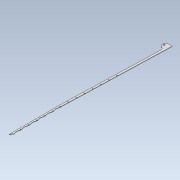
# Autodesk Inventor part: traverse_cote
Saved by Autodesk Inventor 2020 (Build 240168000, 168)
## iProperties
Created: 2020-09-10
Part Number: traverse_cote
Material: Generic
Document SubType Name: Modeling
Designer: Admin
Density: 1 g/cm^3
Appearance: Default
Author: Admin
Autodesk Inventor part; units mm, degrees
ref_plane "YZ Plane" through (0, 0, 0) normal (1, 0, 0) x (0, 1, 0)
ref_plane "XZ Plane" through (0, 0, 0) normal (0, 1, 0) x (-1, 0, 0)
ref_plane "XY Plane" through (0, 0, 0) normal (0, 0, 1) x (1, 0, 0)
sketch "Sketch1" plane through (0, 0, 0) normal (0, 1, 0) x (-1, 0, 0)
  line L0 (0, 0) -> (26.5, 0)
  line L1 (26.5, 0) -> (26.5, -260)
  line L2 (26.5, -260) -> (10, -800)
  line L3 (10, -800) -> (0, -800)
  line L4 (0, 0) -> (0, -10)
  line L5 (0, -10) -> (16.5, -10)
  line L6 (16.5, -10) -> (16.5, -260)
  line L7 (16.5, -260) -> (0, -800)
  dimension "d1" = 26.5
  dimension "d2" = 10
  dimension "d3" = 260
  dimension "d4" = 10
  dimension "d6" = 10
  dimension "d7" = 250
  dimension "d8" = 0
  dimension "d9" = 800
  constraints: 16 end point, 3 perpendicular, 1 coincident, 1 horizontal, 1 parallel, 1 vertical
  measures "d1" distance of L0.start L0.end
  measures "d2" distance of L2.end L3.end
  measures "d3" distance of L0.end L1.end
  measures "d4" distance of L0.start L4.end
  measures "d6" distance between parallel lines of L1 L6
  measures "d7" distance of L5.end L6.end
  measures "d8" horizontal distance of point (0, 0) L3.end
  measures "d9" distance between parallel lines of L0 L3
extrude "Extrusion1" add sketch "Sketch1" along normal mid plane 2
sketch "Sketch2" plane through (0, 1, 0) normal (0, 1, 0) x (1, 0, 0)
  line L0 (-21.5, 50) -> (0, 50)
  line L1 (0, 50) -> (0, 52)
  line L2 (0, 52) -> (-21.5, 52)
  line L3 (-21.5, 52) -> (-21.5, 50)
  line L4 (0, 0) -> (0, 10) projected
  line L5 (0, 10) -> (-16.5, 10) projected
  dimension "d12" = 2
  dimension "d13" = 21.5
  dimension "d14" = 0
  dimension "d16" = 40
  constraints: 8 end point, 2 parallel, 1 horizontal, 1 perpendicular
  measures "d12" distance of L2.end L0.start
  measures "d13" distance of L0.start L0.end
  measures "d14" distance between parallel lines of L4 L1
  measures "d16" distance between parallel lines of L0 L5
extrude "Extrusion2" cut sketch "Sketch2" against normal through all
pattern_linear "Rectangular Pattern1" count 6 spacing 40 along (0, 0, -1) of "Extrusion2"
sketch "Sketch3" plane through (0, 1, 0) normal (0, 1, 0) x (1, 0, 0)
  line L0 (-21.6, 290) -> (0, 290)
  line L1 (0, 290) -> (0, 292)
  line L2 (0, 292) -> (-21.6, 292)
  line L3 (-21.6, 292) -> (-21.6, 290)
  line L4 (0, 0) -> (0, 10) projected
  line L5 (-16.5, 250) -> (-21.5, 250) projected
  line L6 (-19.4, 330) -> (0, 330)
  line L7 (0, 330) -> (0, 332)
  line L8 (0, 332) -> (-19.4, 332)
  line L9 (-19.4, 332) -> (-19.4, 330)
  line L10 (-18.2, 370) -> (0, 370)
  line L11 (0, 370) -> (0, 372)
  line L12 (0, 372) -> (-18.2, 372)
  line L13 (-18.2, 372) -> (-18.2, 370)
  line L14 (-17, 410) -> (0, 410)
  line L15 (0, 410) -> (0, 412)
  line L16 (0, 412) -> (-17, 412)
  line L17 (-17, 412) -> (-17, 410)
  line L18 (-15.8, 450) -> (0, 450)
  line L19 (0, 450) -> (0, 452)
  line L20 (0, 452) -> (-15.8, 452)
  line L21 (-15.8, 452) -> (-15.8, 450)
  line L22 (-14.6, 490) -> (0, 490)
  line L23 (0, 490) -> (0, 492)
  line L24 (0, 492) -> (-14.6, 492)
  line L25 (-14.6, 492) -> (-14.6, 490)
  line L26 (-13.4, 530) -> (0, 530)
  line L27 (0, 530) -> (0, 532)
  line L28 (0, 532) -> (-13.4, 532)
  line L29 (-13.4, 532) -> (-13.4, 530)
  point P0 (-26.5, 250)
  dimension "d22" = 2
  dimension "d23" = 0
  dimension "d24" = 40
  dimension "d25" = 21.6
  dimension "d84" = 40
  dimension "d85" = 2
  dimension "d86" = 0
  dimension "d87" = 19.4
  dimension "d88" = 40
  dimension "d89" = 2
  dimension "d90" = 0
  dimension "d91" = 18.2
  dimension "d92" = 40
  dimension "d93" = 2
  dimension "d94" = 0
  dimension "d95" = 17
  dimension "d96" = 40
  dimension "d97" = 2
  dimension "d98" = 0
  dimension "d99" = 15.8
  dimension "d100" = 40
  dimension "d101" = 2
  dimension "d102" = 0
  dimension "d103" = 14.6
  dimension "d104" = 40
  dimension "d105" = 2
  dimension "d106" = 13.4
  dimension "d107" = 0
  constraints: 56 end point, 14 parallel, 7 horizontal, 7 perpendicular
  measures "d22" distance of L2.end L0.start
  measures "d23" distance from line of L4 L1.end
  measures "d24" distance between parallel lines of L5 L0
  measures "d25" distance of L1.end L2.end
  measures "d84" distance between parallel lines of L6 L0
  measures "d85" distance of L6.end L7.end
  measures "d86" distance between parallel lines of L1 L7
  measures "d87" distance of L6.start L6.end
  measures "d88" distance between parallel lines of L10 L6
  measures "d89" distance of L12.end L10.start
  measures "d90" distance between parallel lines of L7 L11
  measures "d91" distance of L10.start L10.end
  measures "d92" distance between parallel lines of L14 L10
  measures "d93" distance of L16.end L14.start
  measures "d94" distance from line of L10.end L15
  measures "d95" distance of L14.start L14.end
  measures "d96" distance between parallel lines of L18 L14
  measures "d97" distance of L20.end L18.start
  measures "d98" distance between parallel lines of L15 L19
  measures "d99" distance of L18.start L18.end
  measures "d100" distance between parallel lines of L22 L18
  measures "d101" distance of L24.end L22.start
  measures "d102" distance between parallel lines of L23 L19
  measures "d103" distance of L22.start L22.end
  measures "d104" distance between parallel lines of L22 L26
  measures "d105" distance of L28.end L26.start
  measures "d106" distance of L26.start L26.end
  measures "d107" distance from line of L27.end L23
extrude "Extrusion3" cut sketch "Sketch3" against normal through all
sketch "Sketch11" plane through (0, 1, 0) normal (0, 1, 0) x (1, 0, 0)
  line L0 (-22.25, 0) -> (0, 0)
  line L1 (0, 0) -> (0, 10)
  line L2 (0, 10) -> (-22.25, 10)
  line L3 (-22.25, 0) -> (-22.25, 7.5)
  line L4 (-22.25, 7.5) -> (-24.75, 7.5)
  line L5 (-24.75, 7.5) -> (-24.75, 10)
  line L6 (-24.75, 10) -> (-22.25, 10)
  dimension "d108" = 2.5
  dimension "d110" = 2.5
  dimension "d111" = 10
  dimension "d112" = 24.75
  constraints: 14 end point, 4 perpendicular, 1 coincident, 1 horizontal, 1 parallel, 1 point on line, 1 vertical
  measures "d108" distance of L4.end L5.end
  measures "d110" distance of L3.end L4.end
  measures "d111" distance of L0.end L1.end
  measures "d112" distance between parallel lines of L1 L5
extrude "Extrusion11" cut sketch "Sketch11" against normal blind 10
sketch "Sketch12" plane through (0, 1, 0) normal (0, 1, 0) x (1, 0, 0)
  line L0 (-24.75, 7.5) -> (-24.75, 10) projected
  line L1 (-24.75, 7.5) -> (-22.25, 7.5)
  line L2 (-22.25, 7.5) -> (-22.25, 10)
  line L3 (-22.25, 10) -> (-24.75, 10)
  line L4 (-24.75, 10) -> (-24.75, 7.5)
  point P0 (0, 0)
  constraints: 8 end point, 2 parallel, 1 coincident, 1 horizontal, 1 perpendicular
extrude "Extrusion12" add sketch "Sketch12" against normal blind 2
sketch "Sketch13" plane through (0, -1, 0) normal (0, -1, 0) x (1, 0, 0)
  line L0 (-10, -800) -> (-40, -800)
  line L1 (-40, -800) -> (-40, -770)
  line L2 (-40, -770) -> (-10, -770)
  line L3 (-10, -770) -> (-10, -800)
  point P0 (0, 0)
  dimension "d117" = 30
  dimension "d118" = 30
  constraints: 8 end point, 2 parallel, 1 horizontal, 1 perpendicular
  measures "d117" distance of L0.start L0.end
  measures "d118" distance of L2.end L0.start
extrude "Extrusion13" add sketch "Sketch13" against normal blind 2
fillet "Fillet1" radius 15 3 edges at (-40, 0, -770) (-40, 0, -800) (-10.9167, 0, -770)
sketch "Sketch14" plane through (0, -1, 0) normal (0, -1, 0) x (1, 0, 0)
  circle A0 centre (-25, -785) radius 4
  line L0 (-25, -800) -> (0, -800) projected
  point P0 (0, 0)
  dimension "d122" = 8
  dimension "d123" = 25
  dimension "d124" = 15
  constraints: 1 centre point
  measures "d122" diameter of A0
  measures "d123" horizontal distance of A0.centre point (0, 0)
  measures "d124" distance from line of A0.centre L0
extrude "Extrusion14" cut sketch "Sketch14" against normal blind 2
sketch "Sketch15" plane through (0, -1, 0) normal (0, -1, 0) x (1, 0, 0)
  arc A0 (-25.6905, -770.0159) -> (-11.388, -754.5737) centre (-26.381, -755.0318) ccw projected
  arc A1 (-25.6905, -770.0159) -> (-25, -800) centre (-25, -785) ccw projected
  arc A2 (-25.6905, -770.0159) -> (-25, -800) centre (-15.392, -784.7787) ccw
  arc A3 (-25.6905, -770.0159) -> (-25, -800) centre (-25, -785) ccw
  point P0 (0, 0)
  dimension "d127" = 18
  constraints: 5 point on circle, 2 centre point, 1 concentric, 1 equal radius
  measures "d127" radius of A2
extrude "Extrusion15" cut sketch "Sketch15" against normal blind 2
fillet "Fillet2" radius 15 2 edges at (-25, 0, -800) (-25.6905, 0, -770.0159)
sketch "Sketch16" plane through (0, 1, 0) normal (0, 1, 0) x (1, 0, 0)
  arc A0 (-16.5, 45) -> (-16.5, 15) centre (12.8939, 30) ccw
  line L0 (-16.5, 15) -> (-16.5, 45)
  line L1 (-22.25, 10) -> (-16.5, 10) projected
  line L2 (-16.5, 50) -> (-21.5, 50) projected
  line L3 (-16.5, 10) -> (-16.5, 50) projected
  point P0 (0, 0)
  dimension "d131" = 33
  dimension "d132" = 5
  dimension "d133" = 5
  constraints: 2 end point, 2 point on circle, 1 centre point, 1 point on line, 1 vertical
  measures "d131" radius of A0
  measures "d132" distance from line of L0.start L1
  measures "d133" distance from line of L2 L0.end
extrude "Extrusion16" cut sketch "Sketch16" against normal blind 2
pattern_linear "Rectangular Pattern2" count 6 spacing 40 along (0, 0, -1) of "Extrusion16"
body "Solid1"
